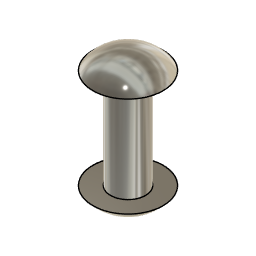
The Rivet (Autodesk Fusion 360 design; units mm, degrees)
Autodesk Fusion 360 part; units mm, degrees
sketch "Sketch1" plane through (0, 0, 0) normal (0, 0, 1) x (1, 0, 0)
  circle A0 centre (0, 0) radius 6
  dimension "d1" = 12
  constraint coincident A0.centre origin
  measures "d1" diameter of A0
extrude "Extrude1" add sketch "Sketch1" along normal mid plane 34 makes body 1
sketch "Sketch2" plane through (0, 0, 0) normal (0, 1, 0) x (1, 0, 0)
  line L0 (0, -17.045) -> (0, -23.045)
  line L1 (0, -23.045) -> (0, -17.045)
  line L2 (0, -17.045) -> (12, -17.045)
  arc A0 (0, -23.045) -> (12, -17.045) centre (0, -8.045) ccw
  dimension "d4" = 6
  dimension "d5" = 12
  dimension "d6" = 15
  constraint vertical L0
  constraint perpendicular L0 L2
  constraint vertical origin L0.start
  measures "d4" distance of L0.start L0.end
  measures "d5" distance of L0.start L2.end
  measures "d6" radius of A0
revolve "Revolve1" add sketch "Sketch2" angle 360 about axis through (0, 0, 0) along (0, 0, -1) separate body makes body 2
mirror "Mirror1" about plane through (0, 0, 0) normal (0, 0, 1) of "Revolve1" makes body 3
